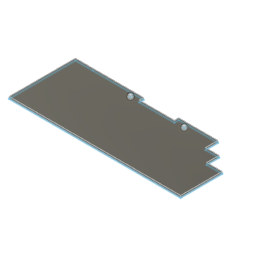
contempt75_case foam 2 v1 (Autodesk Fusion 360 design; units mm, degrees)
Autodesk Fusion 360 part; units mm, degrees
sketch "sketch 290" plane through (0, 0, -8.5) normal (0, 0, 1) x (-1, 0, 0)
  circle A0 centre (-113.5846, 8) radius 1.9
  circle A1 centre (-213.5846, 8) radius 1.9
  line L0 (-294.3039, 46.9884) -> (-294.3039, 24)
  line L1 (-294.3039, 24) -> (-269.2232, 23.9942)
  line L2 (-269.2232, 1) -> (-269.2232, 23.9942)
  line L3 (-269.2232, 1) -> (-196.3771, 1)
  line L4 (-196.3771, 9) -> (-196.3771, 1)
  line L5 (-130.7921, 9) -> (-196.3771, 9)
  line L6 (-130.7921, 1) -> (-130.7921, 9)
  line L7 (-130.7921, 1) -> (-36.7921, 1)
  line L8 (-36.7921, 1) -> (-4, 1)
  line L9 (-4, 1) -> (-4, 124.2856)
  line L10 (-4, 124.2856) -> (-323.1691, 124.2856)
  line L11 (-323.1691, 124.2856) -> (-323.1691, 46.9884)
  line L12 (-294.3039, 46.9884) -> (-323.1691, 46.9884)
extrude "Extrude1" add sketch "sketch 290" along normal blind 3.65
